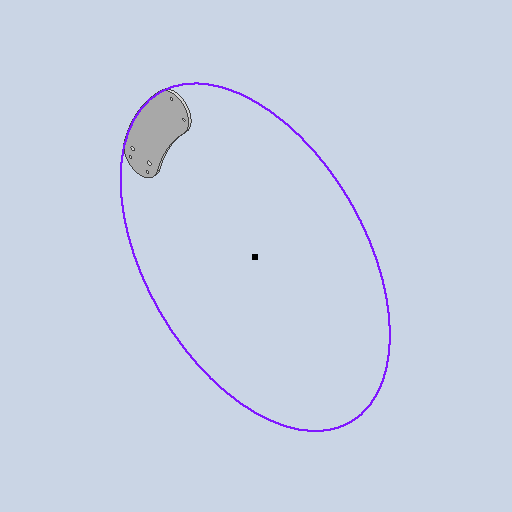
# Autodesk Inventor part: TurretHoodPanel2
Saved by Autodesk Inventor 2022 (Build 260153000, 153)
## iProperties
Created: 2022-01-18
Part Number: TurretHoodPanel2
Material: Generic
Document SubType Name: Modeling
Designer: tagaz
Density: 1 g/cm^3
Appearance: Default
Author: tagaz
Autodesk Inventor part; units mm, degrees
ref_plane "YZ Plane" through (0, 0, 0) normal (1, 0, 0) x (0, 1, 0)
ref_plane "XZ Plane" through (0, 0, 0) normal (0, 1, 0) x (-1, 0, 0)
ref_plane "XY Plane" through (0, 0, 0) normal (0, 0, 1) x (1, 0, 0)
sketch "Sketch1" plane through (0, 0, 0) normal (0, 0, 1) x (1, 0, 0)
  arc A0 (-215.5261, 215.5261) -> (-294.4142, 78.888) centre (0, 0) ccw construction
  arc A1 (-246.957, 246.957) -> (-337.3496, 90.3926) centre (0, 0) ccw
  arc A2 (-184.0953, 184.0953) -> (-251.4788, 67.3835) centre (0, 0) ccw
  arc A3 (-184.0953, 184.0953) -> (-246.957, 246.957) centre (-215.5261, 215.5261) ccw
  arc A4 (-337.3496, 90.3926) -> (-251.4788, 67.3835) centre (-294.4142, 78.888) ccw
  line L0 (0, 0) -> (-294.4142, 78.888) construction
  line L1 (0, 0) -> (294.4142, -78.888) construction
  line L2 (0, 0) -> (-215.5261, 215.5261) construction
  line L3 (0, 0) -> (-111.7396, 0) construction
  line L4 (-246.957, 246.957) -> (-184.0953, 184.0953) construction
  line L5 (-294.4142, 78.888) -> (-251.4788, 67.3835) construction
  line L6 (-337.3496, 90.3926) -> (-294.4142, 78.888) construction
  line L7 (-246.957, 246.957) -> (-215.5261, 215.5261) construction
  line L8 (-184.0953, 184.0953) -> (-215.5261, 215.5261) construction
  arc A5 (-199.8107, 199.8107) -> (-272.9465, 73.1358) centre (0, 0) ccw construction
  arc A6 (-204.3008, 204.3008) -> (-279.0801, 74.7793) centre (0, 0) ccw construction
  arc A7 (-195.3206, 195.3206) -> (-266.8129, 71.4923) centre (0, 0) ccw construction
  arc A8 (-195.3206, 195.3206) -> (-204.3008, 204.3008) centre (-199.8107, 199.8107) ccw construction
  arc A9 (-279.0801, 74.7793) -> (-266.8129, 71.4923) centre (-272.9465, 73.1358) ccw construction
  arc A10 (-231.2416, 231.2416) -> (-315.8819, 84.6403) centre (0, 0) ccw construction
  arc A11 (-235.7317, 235.7317) -> (-322.0155, 86.2838) centre (0, 0) ccw construction
  arc A12 (-226.7515, 226.7515) -> (-309.7483, 82.9968) centre (0, 0) ccw construction
  arc A13 (-226.7515, 226.7515) -> (-235.7317, 235.7317) centre (-231.2416, 231.2416) ccw construction
  arc A14 (-322.0155, 86.2838) -> (-309.7483, 82.9968) centre (-315.8819, 84.6403) ccw construction
  circle A15 centre (-320.9013, 62.9895) radius 3.175
  circle A16 centre (-277.8501, 51.4585) radius 3.175
  circle A17 centre (0, 0) radius 282.575 construction
  circle A18 centre (0, 0) radius 327.025 construction
  circle A19 centre (-183.4894, 214.896) radius 3.175
  circle A20 centre (-215.0012, 246.4139) radius 3.175
  circle A21 centre (-315.8819, 84.6403) radius 4.7625
  circle A22 centre (-272.9465, 73.1358) radius 4.7625
  dimension "d30" = 304.8
  dimension "d31" = 180
  dimension "d32" = 30
  dimension "d33" = 88.9
  dimension "d34" = 45
  dimension "d43" = 12.7
  dimension "d44" = 12.7
  dimension "d45" = 6.35
  dimension "d46" = 6.35
  dimension "d47" = 22.225
  dimension "d48" = 22.225
  dimension "d51" = 6.35
  dimension "d52" = 6.35
  dimension "d53" = 22.225
  dimension "d54" = 22.225
  dimension "d57" = 9.525
  dimension "d58" = 9.525
  constraints: 34 point on circle, 23 centre point, 18 end point, 12 tangent, 7 coincident, 6 collinear, 2 concentric, 2 midpoint, 2 point on line, 1 horizontal, 1 other
  measures "d30" radius of A0
  measures "d31" angle of L0 L1
  measures "d32" angle of L2 L0
  measures "d33" diameter of A3
  measures "d34" angle of L3 L2
  measures "d43" diameter of A8
  measures "d44" diameter of A13
  measures "d45" diameter of A15
  measures "d46" diameter of A16
  measures "d47" distance of A5.end A16.centre
  measures "d48" distance of A10.end A15.centre
  measures "d51" diameter of A19
  measures "d52" diameter of A20
  measures "d53" distance of A20.centre A10.start
  measures "d54" distance of A5.start A19.centre
  measures "d57" diameter of A21
  measures "d58" diameter of A22
extrude "Extrusion1" add sketch "Sketch1" along normal blind 6.35
sketch "Sketch2" plane through (0, 0, 6.35) normal (0, 0, 1) x (1, 0, 0)
  circle A0 centre (0, 0) radius 348.5762
  constraints: 1 centre point, 1 coincident
body "Solid1"
